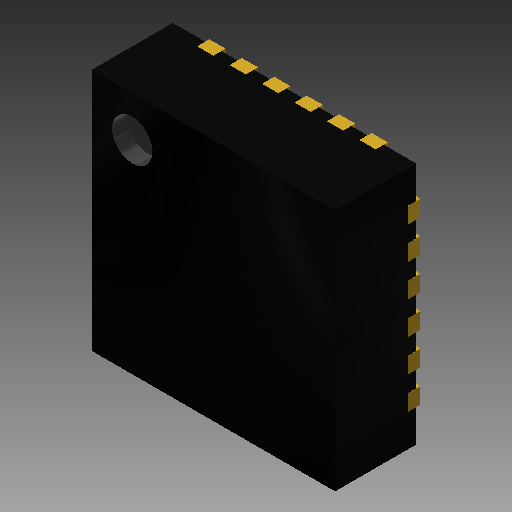
# Autodesk Inventor part: MPU-9250
Saved by Autodesk Inventor 2018 (Build 220112000, 112)
## iProperties
Created: 2016-03-14
Part Number: MPU-9250
Material: Типовые
Document SubType Name: Modeling
Designer: Oleg
Density: 1 g/cm^3
Appearance: По умолчанию
Author: Oleg
Autodesk Inventor part; units mm, degrees
ref_plane "YZ Plane" through (0, 0, 0) normal (1, 0, 0) x (0, 1, 0)
ref_plane "XZ Plane" through (0, 0, 0) normal (0, 1, 0) x (-1, 0, 0)
ref_plane "XY Plane" through (0, 0, 0) normal (0, 0, 1) x (1, 0, 0)
sketch "Эскиз1" plane through (0, 0, 0) normal (0, 0, 1) x (1, 0, 0)
  line L0 (-1.5, 1.5) -> (1.5, 1.5)
  line L1 (1.5, 1.5) -> (1.5, -1.5)
  line L2 (1.5, -1.5) -> (-1.5, -1.5)
  line L3 (-1.5, -1.5) -> (-1.5, 1.5)
  line L4 (-1.5, 1.5) -> (1.5, -1.5) construction
  line L5 (1.5, 1.5) -> (-1.5, -1.5) construction
  point P0 (0, 0)
  point P1 (0, 0)
  dimension "d0" = 3
  constraints: 12 end point, 3 perpendicular, 2 parallel, 1 coincident, 1 horizontal, 1 midpoint
  measures "d0" distance of L0.start L0.end
extrude "Выдавливание1" add sketch "Эскиз1" along normal blind 1
sketch "Эскиз2" plane through (0, 0, 1) normal (0, 0, 1) x (1, 0, 0)
  line L0 (1.5, 1.5) -> (-1.5, 1.5) projected
  line L1 (-1.5, 1.5) -> (-1.5, -1.5) projected
  circle A0 centre (-1, 1) radius 0.25
  point P0 (0, 0)
  dimension "d3" = 0.5
  dimension "d4" = 0.5
  dimension "d5" = 0.5
  constraints: 1 centre point
  measures "d3" diameter of A0
  measures "d4" distance from line of L0 A0.centre
  measures "d5" distance from line of L1 A0.centre
extrude "Выдавливание2" cut sketch "Эскиз2" against normal blind 0.2
sketch "Эскиз3" plane through (0, 0, 0) normal (0, 0, -1) x (-1, 0, 0)
  line L0 (1.5, 1.5) -> (-1.5, 1.5) projected
  line L1 (-1.5, 1.5) -> (-1.5, -1.5) projected
  line L2 (-1.5, -1.5) -> (1.5, -1.5) projected
  line L3 (1.5, -1.5) -> (1.5, 1.5) projected
  line L4 (-1.5, 0) -> (1.5, 0) construction
  line L5 (0, 1.5) -> (0, -1.5) construction
  line L6 (-1.5, 0.3) -> (-1.2, 0.3)
  line L7 (-1.2, 0.3) -> (-1.2, 0.1)
  line L8 (-1.2, 0.1) -> (-1.5, 0.1)
  line L9 (-1.5, 0.1) -> (-1.5, 0.3)
  line L10 (-1.5, 1.1) -> (-1.2, 1.1)
  line L11 (-1.2, 1.1) -> (-1.2, 0.9)
  line L12 (-1.2, 0.9) -> (-1.5, 0.9)
  line L13 (-1.5, 0.9) -> (-1.5, 1.1)
  line L14 (-1.5, 0.7) -> (-1.2, 0.7)
  line L15 (-1.2, 0.7) -> (-1.2, 0.5)
  line L16 (-1.2, 0.5) -> (-1.5, 0.5)
  line L17 (-1.5, 0.5) -> (-1.5, 0.7)
  line L18 (-1.5, -0.1) -> (-1.2, -0.1)
  line L19 (-1.2, -0.1) -> (-1.2, -0.3)
  line L20 (-1.2, -0.3) -> (-1.5, -0.3)
  line L21 (-1.5, -0.3) -> (-1.5, -0.1)
  line L22 (-1.5, -0.5) -> (-1.2, -0.5)
  line L23 (-1.2, -0.5) -> (-1.2, -0.7)
  line L24 (-1.2, -0.7) -> (-1.5, -0.7)
  line L25 (-1.5, -0.7) -> (-1.5, -0.5)
  line L26 (-1.5, -0.9) -> (-1.2, -0.9)
  line L27 (-1.2, -0.9) -> (-1.2, -1.1)
  line L28 (-1.2, -1.1) -> (-1.5, -1.1)
  line L29 (-1.5, -1.1) -> (-1.5, -0.9)
  line L30 (1.5, 0.3) -> (1.2, 0.3)
  line L31 (1.2, 0.3) -> (1.2, 0.1)
  line L32 (1.2, 0.1) -> (1.5, 0.1)
  line L33 (1.5, 0.1) -> (1.5, 0.3)
  line L34 (1.5, 1.1) -> (1.2, 1.1)
  line L35 (1.2, 1.1) -> (1.2, 0.9)
  line L36 (1.2, 0.9) -> (1.5, 0.9)
  line L37 (1.5, 0.9) -> (1.5, 1.1)
  line L38 (1.5, 0.7) -> (1.2, 0.7)
  line L39 (1.2, 0.7) -> (1.2, 0.5)
  line L40 (1.2, 0.5) -> (1.5, 0.5)
  line L41 (1.5, 0.5) -> (1.5, 0.7)
  line L42 (1.5, -0.1) -> (1.2, -0.1)
  line L43 (1.2, -0.1) -> (1.2, -0.3)
  line L44 (1.2, -0.3) -> (1.5, -0.3)
  line L45 (1.5, -0.3) -> (1.5, -0.1)
  line L46 (1.5, -0.5) -> (1.2, -0.5)
  line L47 (1.2, -0.5) -> (1.2, -0.7)
  line L48 (1.2, -0.7) -> (1.5, -0.7)
  line L49 (1.5, -0.7) -> (1.5, -0.5)
  line L50 (1.5, -0.9) -> (1.2, -0.9)
  line L51 (1.2, -0.9) -> (1.2, -1.1)
  line L52 (1.2, -1.1) -> (1.5, -1.1)
  line L53 (1.5, -1.1) -> (1.5, -0.9)
  line L54 (0.1, 1.5) -> (0.3, 1.5)
  line L55 (0.3, 1.5) -> (0.3, 1.2)
  line L56 (0.3, 1.2) -> (0.1, 1.2)
  line L57 (0.1, 1.2) -> (0.1, 1.5)
  line L58 (0.5, 1.5) -> (0.7, 1.5)
  line L59 (0.7, 1.5) -> (0.7, 1.2)
  line L60 (0.7, 1.2) -> (0.5, 1.2)
  line L61 (0.5, 1.2) -> (0.5, 1.5)
  line L62 (0.9, 1.5) -> (1.1, 1.5)
  line L63 (1.1, 1.5) -> (1.1, 1.2)
  line L64 (1.1, 1.2) -> (0.9, 1.2)
  line L65 (0.9, 1.2) -> (0.9, 1.5)
  line L66 (-0.1, 1.5) -> (-0.3, 1.5)
  line L67 (-0.3, 1.5) -> (-0.3, 1.2)
  line L68 (-0.3, 1.2) -> (-0.1, 1.2)
  line L69 (-0.1, 1.2) -> (-0.1, 1.5)
  line L70 (-0.5, 1.5) -> (-0.7, 1.5)
  line L71 (-0.7, 1.5) -> (-0.7, 1.2)
  line L72 (-0.7, 1.2) -> (-0.5, 1.2)
  line L73 (-0.5, 1.2) -> (-0.5, 1.5)
  line L74 (-0.9, 1.5) -> (-1.1, 1.5)
  line L75 (-1.1, 1.5) -> (-1.1, 1.2)
  line L76 (-1.1, 1.2) -> (-0.9, 1.2)
  line L77 (-0.9, 1.2) -> (-0.9, 1.5)
  line L78 (0.1, -1.5) -> (0.3, -1.5)
  line L79 (0.3, -1.5) -> (0.3, -1.2)
  line L80 (0.3, -1.2) -> (0.1, -1.2)
  line L81 (0.1, -1.2) -> (0.1, -1.5)
  line L82 (0.5, -1.5) -> (0.7, -1.5)
  line L83 (0.7, -1.5) -> (0.7, -1.2)
  line L84 (0.7, -1.2) -> (0.5, -1.2)
  line L85 (0.5, -1.2) -> (0.5, -1.5)
  line L86 (0.9, -1.5) -> (1.1, -1.5)
  line L87 (1.1, -1.5) -> (1.1, -1.2)
  line L88 (1.1, -1.2) -> (0.9, -1.2)
  line L89 (0.9, -1.2) -> (0.9, -1.5)
  line L90 (-1.1, -1.2) -> (-0.9, -1.2)
  line L91 (-1.1, -1.5) -> (-1.1, -1.2)
  line L92 (-0.9, -1.5) -> (-1.1, -1.5)
  line L93 (-0.9, -1.2) -> (-0.9, -1.5)
  line L94 (-0.7, -1.2) -> (-0.5, -1.2)
  line L95 (-0.7, -1.5) -> (-0.7, -1.2)
  line L96 (-0.5, -1.5) -> (-0.7, -1.5)
  line L97 (-0.5, -1.2) -> (-0.5, -1.5)
  line L98 (-0.3, -1.5) -> (-0.3, -1.2)
  line L99 (-0.3, -1.2) -> (-0.1, -1.2)
  line L100 (-0.1, -1.2) -> (-0.1, -1.5)
  line L101 (-0.1, -1.5) -> (-0.3, -1.5)
  point P0 (0, 0)
  dimension "d8" = 0.3
  dimension "d9" = 0.2
  dimension "d10" = 0.2
  dimension "d11" = 0.2
  dimension "d12" = 0.2
  dimension "d13" = 0.3
  dimension "d14" = 0.2
  dimension "d15" = 0.2
  dimension "d16" = 0.1
  dimension "d17" = 0.1
  dimension "d18" = 0.2
  dimension "d19" = 0.3
  dimension "d20" = 0.2
  dimension "d21" = 0.2
  dimension "d22" = 0.1
  constraints: 196 end point, 60 symmetric about line, 18 parallel, 12 equal length, 9 horizontal, 9 perpendicular, 3 midpoint, 3 point on line, 8 other
  measures "d8" distance of L6.start L6.end
  measures "d9" distance of L10.end L11.end
  measures "d10" distance between parallel lines of L14 L12
  measures "d11" distance between parallel lines of L6 L16
  measures "d12" distance of L18.end L19.end
  measures "d13" distance of L19.end L20.end
  measures "d14" distance between parallel lines of L22 L20
  measures "d15" distance between parallel lines of L26 L24
  measures "d16" distance between parallel lines of L4 L8
  measures "d17" distance between parallel lines of L4 L18
  measures "d18" distance of L55.end L56.end
  measures "d19" distance of L56.end L54.start
  measures "d20" distance between parallel lines of L61 L55
  measures "d21" distance between parallel lines of L65 L59
  measures "d22" distance between parallel lines of L57 L5
extrude "Выдавливание3" add sketch "Эскиз3" along normal blind 0.05 contours L63 L64 L65 L0 | L3 L36 L35 L34 | L59 L60 L61 L0 | L3 L40 L39 L38 | L55 L56 L57 L0 | L3 L32 L31 L30 | L69 L68 L67 L0 | L3 L44 L43 L42 | L73 L72 L71 L0 | L3 L48 L47 L46 | L77 L76 L75 L0 | L3 L52 L51 L50 | L10 L11 L12 L1 | L2 L89 L88 L87 | L14 L15 L16 L1 | L2 L85 L84 L83 | L6 L7 L8 L1 | L2 L81 L80 L79 | L18 L19 L20 L1 | L2 L98 L99 L100 | L22 L23 L24 L1 | L2 L95 L94 L97 | L26 L27 L28 L1 | L2 L91 L90 L93
sketch "Эскиз4" plane through (-1.5, -1.5, 1) normal (0, -1, 0) x (1, 0, 0)
  line L0 (0.4, -1.05) -> (0.6, -1.05)
  line L1 (0.6, -1.05) -> (0.6, -0.9)
  line L2 (0.6, -0.9) -> (0.4, -0.9)
  line L3 (0.4, -0.9) -> (0.4, -1.05)
  line L4 (1, -1.05) -> (0.8, -1.05)
  line L5 (0.8, -1.05) -> (0.8, -0.9)
  line L6 (0.8, -0.9) -> (1, -0.9)
  line L7 (1, -0.9) -> (1, -1.05)
  line L8 (1.4, -1.05) -> (1.2, -1.05)
  line L9 (1.2, -1.05) -> (1.2, -0.9)
  line L10 (1.2, -0.9) -> (1.4, -0.9)
  line L11 (1.4, -0.9) -> (1.4, -1.05)
  line L12 (1.8, -1.05) -> (1.6, -1.05)
  line L13 (1.6, -1.05) -> (1.6, -0.9)
  line L14 (1.6, -0.9) -> (1.8, -0.9)
  line L15 (1.8, -0.9) -> (1.8, -1.05)
  line L16 (2.2, -1.05) -> (2, -1.05)
  line L17 (2, -1.05) -> (2, -0.9)
  line L18 (2, -0.9) -> (2.2, -0.9)
  line L19 (2.2, -0.9) -> (2.2, -1.05)
  line L20 (2.6, -1.05) -> (2.4, -1.05)
  line L21 (2.4, -1.05) -> (2.4, -0.9)
  line L22 (2.4, -0.9) -> (2.6, -0.9)
  line L23 (2.6, -0.9) -> (2.6, -1.05)
  point P0 (1.5, -1)
  dimension "d25" = 0.15
  dimension "d26" = 0.2
  constraints: 48 end point, 12 parallel, 9 equal length, 6 horizontal, 6 perpendicular
  measures "d25" distance of L20.end L21.end
  measures "d26" distance of L21.end L22.end
extrude "Выдавливание4" add sketch "Эскиз4" along normal blind 0.001
sketch "Эскиз5" plane through (1.5, -1.5, 1) normal (1, 0, 0) x (0, 0, -1)
  line L0 (1.05, 0.4) -> (0.9, 0.4)
  line L1 (0.9, 0.4) -> (0.9, 0.6)
  line L2 (0.9, 0.6) -> (1.05, 0.6)
  line L3 (1.05, 0.6) -> (1.05, 0.4)
  line L4 (1.05, 0.8) -> (0.9, 0.8)
  line L5 (0.9, 0.8) -> (0.9, 1)
  line L6 (0.9, 1) -> (1.05, 1)
  line L7 (1.05, 1) -> (1.05, 0.8)
  line L8 (1.05, 1.2) -> (0.9, 1.2)
  line L9 (0.9, 1.2) -> (0.9, 1.4)
  line L10 (0.9, 1.4) -> (1.05, 1.4)
  line L11 (1.05, 1.4) -> (1.05, 1.2)
  line L12 (1.05, 1.6) -> (0.9, 1.6)
  line L13 (0.9, 1.6) -> (0.9, 1.8)
  line L14 (0.9, 1.8) -> (1.05, 1.8)
  line L15 (1.05, 1.8) -> (1.05, 1.6)
  line L16 (1.05, 2) -> (0.9, 2)
  line L17 (0.9, 2) -> (0.9, 2.2)
  line L18 (0.9, 2.2) -> (1.05, 2.2)
  line L19 (1.05, 2.2) -> (1.05, 2)
  line L20 (1.05, 2.4) -> (0.9, 2.4)
  line L21 (0.9, 2.4) -> (0.9, 2.6)
  line L22 (0.9, 2.6) -> (1.05, 2.6)
  line L23 (1.05, 2.6) -> (1.05, 2.4)
  point P0 (1, 1.5)
  dimension "d29" = 0.2
  dimension "d30" = 0.15
  constraints: 48 end point, 12 parallel, 9 equal length, 6 horizontal, 6 perpendicular
  measures "d29" distance of L20.end L21.end
  measures "d30" distance of L21.end L22.end
extrude "Выдавливание5" add sketch "Эскиз5" along normal blind 0.001
sketch "Эскиз6" plane through (-1.5, 1.5, 1) normal (0, 1, 0) x (1, 0, 0)
  line L0 (2.6, 1.05) -> (2.4, 1.05)
  line L1 (2.4, 1.05) -> (2.4, 0.9)
  line L2 (2.4, 0.9) -> (2.6, 0.9)
  line L3 (2.6, 0.9) -> (2.6, 1.05)
  line L4 (2.2, 1.05) -> (2, 1.05)
  line L5 (2, 1.05) -> (2, 0.9)
  line L6 (2, 0.9) -> (2.2, 0.9)
  line L7 (2.2, 0.9) -> (2.2, 1.05)
  line L8 (1.8, 1.05) -> (1.6, 1.05)
  line L9 (1.6, 1.05) -> (1.6, 0.9)
  line L10 (1.6, 0.9) -> (1.8, 0.9)
  line L11 (1.8, 0.9) -> (1.8, 1.05)
  line L12 (1.4, 1.05) -> (1.2, 1.05)
  line L13 (1.2, 1.05) -> (1.2, 0.9)
  line L14 (1.2, 0.9) -> (1.4, 0.9)
  line L15 (1.4, 0.9) -> (1.4, 1.05)
  line L16 (1, 1.05) -> (0.8, 1.05)
  line L17 (0.8, 1.05) -> (0.8, 0.9)
  line L18 (0.8, 0.9) -> (1, 0.9)
  line L19 (1, 0.9) -> (1, 1.05)
  line L20 (0.6, 1.05) -> (0.4, 1.05)
  line L21 (0.4, 1.05) -> (0.4, 0.9)
  line L22 (0.4, 0.9) -> (0.6, 0.9)
  line L23 (0.6, 0.9) -> (0.6, 1.05)
  point P0 (1.5, 1)
  dimension "d33" = 0.15
  dimension "d34" = 0.2
  constraints: 48 end point, 12 parallel, 10 equal length, 6 horizontal, 6 perpendicular
  measures "d33" distance of L2.end L0.start
  measures "d34" distance of L1.end L2.end
extrude "Выдавливание6" add sketch "Эскиз6" along normal blind 0.001
sketch "Эскиз7" plane through (-1.5, -1.5, 1) normal (-1, 0, 0) x (0, 0, 1)
  line L0 (-1.05, 2.6) -> (-0.9, 2.6)
  line L1 (-0.9, 2.6) -> (-0.9, 2.4)
  line L2 (-0.9, 2.4) -> (-1.05, 2.4)
  line L3 (-1.05, 2.4) -> (-1.05, 2.6)
  line L4 (-1.05, 2.2) -> (-0.9, 2.2)
  line L5 (-0.9, 2.2) -> (-0.9, 2)
  line L6 (-0.9, 2) -> (-1.05, 2)
  line L7 (-1.05, 2) -> (-1.05, 2.2)
  line L8 (-1.05, 1.8) -> (-0.9, 1.8)
  line L9 (-0.9, 1.8) -> (-0.9, 1.6)
  line L10 (-0.9, 1.6) -> (-1.05, 1.6)
  line L11 (-1.05, 1.6) -> (-1.05, 1.8)
  line L12 (-1.05, 1.4) -> (-0.9, 1.4)
  line L13 (-0.9, 1.4) -> (-0.9, 1.2)
  line L14 (-0.9, 1.2) -> (-1.05, 1.2)
  line L15 (-1.05, 1.2) -> (-1.05, 1.4)
  line L16 (-1.05, 1) -> (-0.9, 1)
  line L17 (-0.9, 1) -> (-0.9, 0.8)
  line L18 (-0.9, 0.8) -> (-1.05, 0.8)
  line L19 (-1.05, 0.8) -> (-1.05, 1)
  line L20 (-1.05, 0.6) -> (-0.9, 0.6)
  line L21 (-0.9, 0.6) -> (-0.9, 0.4)
  line L22 (-0.9, 0.4) -> (-1.05, 0.4)
  line L23 (-1.05, 0.4) -> (-1.05, 0.6)
  point P0 (-1, 1.5)
  dimension "d37" = 0.15
  dimension "d38" = 0.2
  constraints: 48 end point, 12 parallel, 10 equal length, 6 horizontal, 6 perpendicular
  measures "d37" distance of L0.start L0.end
  measures "d38" distance of L0.end L1.end
extrude "Выдавливание7" add sketch "Эскиз7" along normal blind 0.001
